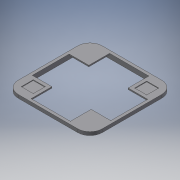
# Autodesk Inventor part: Wandhalterung
Saved by Autodesk Inventor 2016 SP2 (Build 200236200, 236)
## iProperties
Created: 2018-06-26
Part Number: Wandhalterung
Material: Generisch
Document SubType Name: Modeling
Designer: Nils
Density: 1 g/cm^3
Appearance: Vorgabe
Author: Nils
Autodesk Inventor part; units mm, degrees
ref_plane "YZ Plane" through (0, 0, 0) normal (1, 0, 0) x (0, 1, 0)
ref_plane "XZ Plane" through (0, 0, 0) normal (0, 1, 0) x (-1, 0, 0)
ref_plane "XY Plane" through (0, 0, 0) normal (0, 0, 1) x (1, 0, 0)
sketch "Skizze1" plane through (0, 0, 0) normal (0, 0, 1) x (1, 0, 0)
  line L0 (32.9869, 99.2902) -> (32.9869, 40.1902) construction
  arc A0 (22.9869, 30.1902) -> (32.9869, 40.1902) centre (22.9869, 40.1902) ccw construction
  line L1 (22.9869, 30.1902) -> (-36.1131, 30.1902) construction
  arc A1 (-46.1131, 40.1902) -> (-36.1131, 30.1902) centre (-36.1131, 40.1902) ccw construction
  line L2 (-46.1131, 40.1902) -> (-46.1131, 99.2902) construction
  arc A2 (-36.1131, 109.2902) -> (-46.1131, 99.2902) centre (-36.1131, 99.2902) ccw construction
  line L3 (-36.1131, 109.2902) -> (22.9869, 109.2902) construction
  arc A3 (32.9869, 99.2902) -> (22.9869, 109.2902) centre (22.9869, 99.2902) ccw construction
  arc A4 (-38.6131, 111.7902) -> (-48.6131, 101.7902) centre (-38.6131, 101.7902) ccw construction
  line L4 (-48.6131, 101.7902) -> (-48.6131, 37.6902) construction
  arc A5 (-48.6131, 37.6902) -> (-38.6131, 27.6902) centre (-38.6131, 37.6902) ccw construction
  line L5 (-38.6131, 27.6902) -> (25.4869, 27.6902) construction
  arc A6 (25.4869, 27.6902) -> (35.4869, 37.6902) centre (25.4869, 37.6902) ccw construction
  line L6 (35.4869, 37.6902) -> (35.4869, 101.7902) construction
  arc A7 (35.4869, 101.7902) -> (25.4869, 111.7902) centre (25.4869, 101.7902) ccw construction
  line L7 (25.4869, 111.7902) -> (-38.6131, 111.7902) construction
  arc A8 (-38.6131, 111.9702) -> (-48.7931, 101.7902) centre (-38.6131, 101.7902) ccw
  line L8 (-48.7931, 101.7902) -> (-48.7931, 37.6902)
  arc A9 (-48.7931, 37.6902) -> (-38.6131, 27.5102) centre (-38.6131, 37.6902) ccw
  line L9 (-38.6131, 27.5102) -> (25.4869, 27.5102)
  arc A10 (25.4869, 27.5102) -> (35.6669, 37.6902) centre (25.4869, 37.6902) ccw
  line L10 (35.6669, 37.6902) -> (35.6669, 101.7902)
  arc A11 (35.6669, 101.7902) -> (25.4869, 111.9702) centre (25.4869, 101.7902) ccw
  line L11 (25.4869, 111.9702) -> (-38.6131, 111.9702)
  arc A12 (-38.6131, 114.9702) -> (-51.7931, 101.7902) centre (-38.6131, 101.7902) ccw
  line L12 (-38.6131, 114.9702) -> (25.4869, 114.9702)
  arc A13 (38.6669, 101.7902) -> (25.4869, 114.9702) centre (25.4869, 101.7902) ccw
  line L13 (38.6669, 101.7902) -> (38.6669, 37.6902)
  arc A14 (25.4869, 24.5102) -> (38.6669, 37.6902) centre (25.4869, 37.6902) ccw
  line L14 (25.4869, 24.5102) -> (-38.6131, 24.5102)
  arc A15 (-51.7931, 37.6902) -> (-38.6131, 24.5102) centre (-38.6131, 37.6902) ccw
  line L15 (-51.7931, 37.6902) -> (-51.7931, 101.7902)
  line L16 (12.5869, 111.9702) -> (12.5869, 87.8902)
  line L17 (12.5869, 87.8902) -> (35.6669, 87.8902)
  circle A16 centre (24.5869, 99.8902) radius 5.075 construction
  circle A17 centre (-37.7131, 39.5902) radius 5.075 construction
  line L18 (-48.7931, 51.5902) -> (-25.7131, 51.5902)
  line L19 (-25.7131, 51.5902) -> (-25.7131, 27.5102)
  point P0 (0, 0)
  dimension "d0" = 0.18
  dimension "d1" = 3
  dimension "d2" = 12
  dimension "d3" = 12
  dimension "d4" = 12
  dimension "d5" = 12
  constraints: 24 end point, 16 point on circle, 8 centre point, 4 perpendicular, 4 point on line, 14 other
  measures "d0" distance between parallel lines of L7 L11
  measures "d1" radial gap between concentric circles of A8 A12
  measures "d2" distance from line of L16 A16.centre
  measures "d3" distance from line of A16.centre L17
  measures "d4" distance from line of L18 A17.centre
  measures "d5" distance from line of A17.centre L19
extrude "Extrusion1" add sketch "Skizze1" along normal blind 5
chamfer "Fase1" distance 2 angle 35 8 edges at (34.8066, 111.1099, 0) (38.6669, 69.7402, 0) (34.8066, 28.3705, 0) (-6.5631, 24.5102, 0) (-47.9328, 28.3705, 0) (-51.7931, 69.7402, 0) (-47.9328, 111.1099, 0) (-6.5631, 114.9702, 0) measured on face at (-12.9464, 25.5102, 0)
sketch "Skizze2" plane through (0, 0, 5) normal (0, 0, 1) x (1, 0, 0)
  circle A0 centre (-37.7131, 39.5902) radius 5.075 construction
  circle A1 centre (24.5869, 99.8902) radius 5.075 construction
  line L0 (-48.7931, 37.6902) -> (-48.7931, 101.7902) projected
  line L1 (-48.7931, 49.5902) -> (-27.7131, 49.5902)
  line L2 (-27.7131, 49.5902) -> (-27.7131, 27.5102)
  line L3 (-38.6131, 27.5102) -> (25.4869, 27.5102) projected
  arc A2 (-48.7931, 37.6902) -> (-38.6131, 27.5102) centre (-38.6131, 37.6902) ccw projected
  line L4 (35.6669, 101.7902) -> (35.6669, 37.6902) projected
  arc A3 (35.6669, 101.7902) -> (25.4869, 111.9702) centre (25.4869, 101.7902) ccw projected
  line L5 (-38.6131, 111.9702) -> (25.4869, 111.9702) projected
  line L6 (25.4869, 111.9702) -> (-38.6131, 111.9702) projected
  line L7 (14.5869, 111.9702) -> (14.5869, 89.8902)
  line L8 (14.5869, 89.8902) -> (35.6669, 89.8902)
  arc A4 (-38.6131, 111.9702) -> (-48.7931, 101.7902) centre (-38.6131, 101.7902) ccw projected
  arc A5 (25.4869, 27.5102) -> (35.6669, 37.6902) centre (25.4869, 37.6902) ccw projected
  line L9 (14.5869, 27.5102) -> (14.5869, 49.5902)
  line L10 (14.5869, 49.5902) -> (35.6669, 49.5902)
  line L11 (35.6669, 37.6902) -> (35.6669, 101.7902) projected
  line L12 (-48.7931, 89.8902) -> (-27.7131, 89.8902)
  line L13 (-27.7131, 89.8902) -> (-27.7131, 111.9702)
  point P0 (0, 0)
  dimension "d11" = 10
  dimension "d12" = 10
  dimension "d13" = 10
  dimension "d14" = 10
  constraints: 16 end point, 8 point on line, 6 perpendicular, 4 collinear, 2 horizontal
  measures "d11" distance from line of A1.centre L7
  measures "d12" distance from line of L8 A1.centre
  measures "d13" distance from line of L1 A0.centre
  measures "d14" distance from line of L2 A0.centre
extrude "Extrusion2" add sketch "Skizze2" against normal blind 1.4 contours L0 L1 L2 L3 A2 | L0 A4 L5 L13 L12 | L9 L10 L4 A5 L3 | L5 A3 L4 L8 L7
sketch "Skizze3" plane through (0, 0, 5) normal (0, 0, 1) x (1, 0, 0)
  circle A0 centre (-37.7131, 39.5902) radius 5.075 construction
  circle A1 centre (24.5869, 99.8902) radius 4.075 construction
  line L0 (18.0869, 93.3902) -> (31.0869, 93.3902)
  line L1 (31.0869, 93.3902) -> (31.0869, 106.3902)
  line L2 (31.0869, 106.3902) -> (18.0869, 106.3902)
  line L3 (18.0869, 106.3902) -> (18.0869, 93.3902)
  line L4 (18.0869, 93.3902) -> (31.0869, 106.3902) construction
  line L5 (31.0869, 93.3902) -> (18.0869, 106.3902) construction
  line L6 (-44.2131, 33.0902) -> (-31.2131, 33.0902)
  line L7 (-31.2131, 33.0902) -> (-31.2131, 46.0902)
  line L8 (-31.2131, 46.0902) -> (-44.2131, 46.0902)
  line L9 (-44.2131, 46.0902) -> (-44.2131, 33.0902)
  line L10 (-44.2131, 33.0902) -> (-31.2131, 46.0902) construction
  line L11 (-31.2131, 33.0902) -> (-44.2131, 46.0902) construction
  point P0 (0, 0)
  dimension "d17" = 13
  dimension "d18" = 13
  dimension "d19" = 13
  dimension "d20" = 13
  constraints: 24 end point, 4 midpoint, 4 parallel, 2 horizontal, 2 perpendicular
  measures "d17" distance of L2.end L1.end
  measures "d18" distance of L1.end L0.end
  measures "d19" distance of L8.end L7.end
  measures "d20" distance of L7.end L6.end
extrude "Extrusion3" cut sketch "Skizze3" against normal blind 0.8
equation "\"d2\" = d3"
equation "\"d4\" = d3"
equation "\"d5\" = d4"
